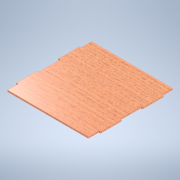
# Autodesk Inventor part: ControlPanelPlate_V1-01
Saved by Autodesk Inventor 2022.2 (Build 262287000, 287)
## iProperties
Created: 2022-11-17
Part Number: ControlPanelPlate_V1-01
Material: Generic
Document SubType Name: Modeling
Designer: jaege
Density: 1 g/cm^3
Appearance: Red Oak - Natural Low Gloss
Author: jaege
Autodesk Inventor part; units mm, degrees
ref_plane "YZ Plane" through (0, 0, 0) normal (1, 0, 0) x (0, 1, 0)
ref_plane "XZ Plane" through (0, 0, 0) normal (0, 1, 0) x (-1, 0, 0)
ref_plane "XY Plane" through (0, 0, 0) normal (0, 0, 1) x (1, 0, 0)
sketch "Sketch1" plane through (0, 0, 0) normal (0, 1, 0) x (-1, 0, 0)
  line L0 (96, -100) -> (-96, -100)
  line L1 (-96, -100) -> (-96, 100)
  line L2 (-96, 100) -> (96, 100)
  line L3 (96, 100) -> (96, -100)
  line L4 (96, -100) -> (-96, 100) construction
  line L5 (-96, -100) -> (96, 100) construction
  line L6 (96, -75) -> (100, -75)
  line L7 (100, -75) -> (100, -25)
  line L8 (100, -25) -> (96, -25)
  line L9 (96, -25) -> (96, -75)
  line L10 (96, -25) -> (100, -25)
  line L11 (100, -25) -> (100, 25)
  line L12 (100, 25) -> (96, 25)
  line L13 (96, 25) -> (96, -25)
  line L14 (96, 25) -> (100, 25)
  line L15 (100, 25) -> (100, 75)
  line L16 (100, 75) -> (96, 75)
  line L17 (96, 75) -> (96, 25)
  line L18 (-96, -75) -> (-100, -75)
  line L19 (-100, -75) -> (-100, -25)
  line L20 (-100, -25) -> (-96, -25)
  line L21 (-96, -25) -> (-96, -75)
  line L22 (-96, -25) -> (-100, -25)
  line L23 (-100, -25) -> (-100, 25)
  line L24 (-100, 25) -> (-96, 25)
  line L25 (-96, 25) -> (-96, -25)
  line L26 (-96, 25) -> (-100, 25)
  line L27 (-100, 25) -> (-100, 75)
  line L28 (-100, 75) -> (-96, 75)
  line L29 (-96, 75) -> (-96, 25)
  point P0 (0, 0)
  point P1 (98, -75)
  point P2 (-98, -75)
  dimension "d0" = 192
  dimension "d1" = 200
  dimension "d2" = 4
  dimension "d3" = 50
  dimension "d4" = 4
  dimension "d5" = 50
  dimension "d6" = 4
  dimension "d7" = 50
  dimension "d8" = 4
  dimension "d9" = 50
  dimension "d10" = 4
  dimension "d11" = 50
  dimension "d12" = 4
  dimension "d13" = 50
  dimension "d14" = 25
  dimension "d15" = 25
  constraints: 60 end point, 14 parallel, 7 horizontal, 7 perpendicular, 4 midpoint, 2 point on line
  measures "d0" distance of L1.end L2.end
  measures "d1" distance of L0.end L1.end
  measures "d2" distance of L8.end L7.end
  measures "d3" distance of L7.end L6.end
  measures "d4" distance of L12.end L11.end
  measures "d5" distance of L11.end L10.end
  measures "d6" distance of L16.end L15.end
  measures "d7" distance of L15.end L14.end
  measures "d8" distance of L19.end L20.end
  measures "d9" distance of L18.end L19.end
  measures "d10" distance of L23.end L24.end
  measures "d11" distance of L22.end L23.end
  measures "d12" distance of L27.end L28.end
  measures "d13" distance of L26.end L27.end
  measures "d14" distance from line of L0 point (98, -75)
  measures "d15" distance from line of L0 point (-98, -75)
extrude "Extrusion1" add sketch "Sketch1" along normal blind 4 contours L0 L1 L2 L3 | L3 L8 L7 L6 | L18 L19 L20 L1 | L3 L16 L15 L12 | L24 L27 L28 L1
body "Solid1"
